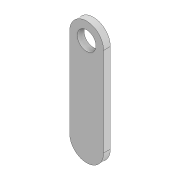
# Autodesk Inventor part: SecondPendulum
Saved by Autodesk Inventor 2020 (Build 240168000, 168)
## iProperties
Created: 2021-06-21
Part Number: SecondPendulum
Material: Generic
Document SubType Name: Modeling
Designer: Aidan Lee
Density: 1 g/cm^3
Appearance: Default
Author: Aidan Lee
Autodesk Inventor part; units mm, degrees
ref_plane "YZ Plane" through (0, 0, 0) normal (1, 0, 0) x (0, 1, 0)
ref_plane "XZ Plane" through (0, 0, 0) normal (0, 1, 0) x (-1, 0, 0)
ref_plane "XY Plane" through (0, 0, 0) normal (0, 0, 1) x (1, 0, 0)
sketch "Sketch1" plane through (0, 0, 0) normal (0, 0, 1) x (1, 0, 0)
  line L0 (0, 0) -> (220, 0) construction
  line L1 (220, 0) -> (220, 9) construction
  line L2 (220, 9) -> (0, 9) construction
  line L3 (0, 9) -> (0, 0) construction
  line L4 (0, 9) -> (90.94, 295.0593) construction
  line L5 (129.06, 295.0593) -> (220, 9) construction
  circle A0 centre (110, 289) radius 11 construction
  line L6 (96.1101, 281.616) -> (103.5522, 305.0259) construction
  arc A1 (129.06, 295.0593) -> (90.94, 295.0593) centre (110, 289) ccw construction
  line L7 (99, 275.5567) -> (99, 269.1274) construction
  line L8 (110, 289) -> (110, 144) construction
  line L9 (130, 289) -> (130, 144) construction
  line L10 (90, 144) -> (90, 289) construction
  arc A2 (130, 289) -> (90, 289) centre (110, 289) ccw construction
  arc A3 (90, 144) -> (130, 144) centre (110, 144) ccw construction
  line L11 (290, 144) -> (290, 249) construction
  line L12 (310, 144) -> (310, 249) construction
  line L13 (270, 249) -> (270, 144) construction
  arc A4 (270, 144) -> (310, 144) centre (290, 144) ccw construction
  arc A5 (310, 249) -> (270, 249) centre (290, 249) ccw construction
  arc A6 (90, 289) -> (130, 289) centre (110, 289) ccw construction
  line L14 (98.9216, 269) -> (121.0784, 269) construction
  line L15 (209.0249, 269) -> (370.9751, 269) construction
  line L16 (209.0249, 144) -> (370.9751, 144) construction
  line L17 (290, 144) -> (290, 39) construction
  line L18 (310, 144) -> (310, 39)
  line L19 (270, 39) -> (270, 144)
  arc A7 (310, 144) -> (270, 144) centre (290, 144) ccw
  arc A8 (270, 39) -> (310, 39) centre (290, 39) ccw
  line L20 (209.0249, 19) -> (370.9751, 19) construction
  circle A9 centre (110, 289) radius 11 construction
  circle A10 centre (110, 144) radius 11 construction
  circle A11 centre (290, 144) radius 11
  circle A12 centre (290, 39) radius 11
  point P0 (110, 0)
  point P1 (110, 216.5)
  point P2 (110, 309)
  point P3 (290, 196.5)
  point P4 (110, 269)
  point P5 (110, 269)
  point P6 (290, 269)
  dimension "d0" = 9
  dimension "d1" = 220
  dimension "d2" = 22
  dimension "d3" = 280
  dimension "d4" = 9
  dimension "d7" = 40
  dimension "d8" = 40
  dimension "pendgap" = 0
  dimension "abovethefloor" = 10
  dimension "d11" = 105
  dimension "d12" = 145
  dimension "d14" = 22
  dimension "d18" = 22
  dimension "d19" = 22
  dimension "d20" = 50
  constraints: 48 end point, 19 point on circle, 14 tangent, 13 centre point, 7 coincident, 6 midpoint, 5 parallel, 5 symmetric about line, 4 horizontal, 3 vertical, 2 vertical alignment, 1 concentric, 1 horizontal alignment, 1 perpendicular, 2 other
  measures "d0" distance of L2.end L0.start
  measures "d1" distance of L0.start L0.end
  measures "d2" diameter of A0
  measures "d3" distance from line of L2 A0.centre
  measures "d4" distance between parallel lines of L4 L6
  measures "d7" distance between parallel lines of L9 L10
  measures "d8" distance between parallel lines of L12 L13
  measures "pendgap" distance between parallel lines of L15 L14
  measures "abovethefloor" distance between parallel lines of L2 L20
  measures "d11" distance of L11.start L17.end
  measures "d12" distance of A0.centre L8.end
  measures "d14" diameter of A10
  measures "d18" diameter of A11
  measures "d19" diameter of A12
  measures "d20" distance between parallel lines of L13 L1
extrude "Extrusion3" add sketch "Sketch1" along normal blind 8 contours L18 A8 L19 A7 | A12
body "Solid3"
